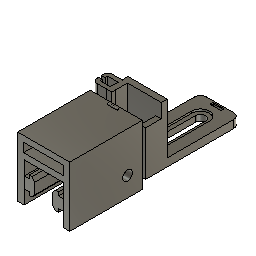
Sensor_Support (Autodesk Fusion 360 design; units mm, degrees)
Autodesk Fusion 360 part; units mm, degrees
sketch "Esquisse1" plane through (0, 0, 0) normal (0, 0, 1) x (1, 0, 0)
  line L0 (0, 80) -> (0, -6.3898) construction
  line L1 (-15, 30) -> (6, 30) construction
  line L2 (-7.25, 0) -> (7.25, 0)
  line L3 (7.25, 0) -> (7.25, -6)
  line L4 (-7.25, -6) -> (-7.25, 0)
  line L5 (-5.5, -1) -> (5.5, -1)
  line L6 (5.5, -1) -> (5.5, -6)
  line L7 (5.5, -6) -> (-5.5, -6)
  line L8 (-5.5, -6) -> (-5.5, -1)
  line L9 (5.5, -6) -> (7.25, -6)
  line L10 (7.25, -6) -> (-5.5, -6)
  line L11 (-7.25, -6) -> (-5.5, -6)
  line L12 (-10, 0) -> (-10, 37)
  line L13 (-7, 40) -> (7, 40)
  arc A0 (4.5, 30) -> (-4.5, 30) centre (0, 30) ccw
  arc A1 (2.5, 30) -> (-2.5, 30) centre (0, 30) ccw
  line L14 (-13, 20) -> (15, 20) construction
  line L15 (-13, 10) -> (15, 10) construction
  arc A2 (-4.5, 10) -> (4.5, 10) centre (0, 10) ccw
  arc A3 (-2.5, 10) -> (2.5, 10) centre (0, 10) ccw
  line L16 (-4.5, 30) -> (-4.5, 10)
  line L17 (-2.5, 30) -> (-2.5, 10)
  line L18 (2.5, 30) -> (2.5, 10)
  line L19 (4.5, 30) -> (4.5, 10)
  line L20 (-19.75, -1.5) -> (-19.75, -9) construction
  line L21 (-15.265, -2) -> (-12, -2)
  line L22 (-10, -8) -> (-14.75, -8)
  line L23 (-14.7654, 0) -> (-10, 0)
  line L24 (-17.25, -3.35) -> (-15.265, -3.35)
  line L25 (-15.25, -4.7238) -> (-17.25, -4.7238)
  line L26 (-15.265, -3.35) -> (-15.265, -2)
  line L27 (-17.25, -5.5) -> (-17.25, -4.7238)
  line L28 (-17.25, -3.35) -> (-17.265, -2.5467)
  arc A4 (-14.7654, 0) -> (-17.265, -2.5467) centre (-14.7654, -2.5) ccw
  arc A5 (-17.25, -5.5) -> (-14.75, -8) centre (-14.75, -5.5) ccw
  line L29 (-12, -2) -> (-10, -2)
  line L30 (-10, -2) -> (-10, -6)
  line L31 (-10, -6) -> (-15.25, -6)
  line L32 (-15.25, -6) -> (-15.25, -4.7238)
  line L33 (-13, -4.0369) -> (-21, -4.0369) construction
  line L34 (10, -8) -> (-10, -8)
  line L35 (10, 37) -> (10, -8)
  line L36 (10, 3) -> (-10, 3)
  arc A6 (-7, 40) -> (-10, 37) centre (-7, 37) ccw
  arc A7 (10, 37) -> (7, 40) centre (7, 37) ccw
  line L37 (-2.5, 39) -> (2.5, 39)
  line L38 (2.5, 39) -> (2.5, 38)
  line L39 (2.5, 38) -> (-2.5, 38)
  line L40 (-2.5, 38) -> (-2.5, 39)
  dimension "d49" = 11
  dimension "d50" = 5
  dimension "d51" = 1
  dimension "d52" = 14.5
  dimension "d67" = 30
  dimension "d68" = 5
  dimension "d86" = 10
  dimension "d87" = 2
  dimension "d100" = 2.5
  dimension "d101" = 2.5
  dimension "d108" = 2
  dimension "d109" = 2
  dimension "d111" = 1.3738
  dimension "d112" = 2
  dimension "d113" = 2
  dimension "d114" = 5.25
  dimension "d115" = 4
  dimension "d117" = 1.2762
  dimension "d132" = 2
  dimension "d133" = 5.265
  dimension "d135" = 48
  dimension "d136" = 20
  dimension "d137" = 2.75
  dimension "d140" = 3
  dimension "d153" = 3
  dimension "d154" = 1
  dimension "d155" = 1
  dimension "d156" = 5
  constraint perpendicular L0 L1
  constraint horizontal L2
  constraint vertical L3
  constraint vertical L4
  constraint symmetric L0 L3 L4
  constraint horizontal L5
  constraint vertical L6
  constraint horizontal L7
  constraint vertical L8
  constraint symmetric L0 L6 L8
  constraint coincident origin L0
  constraint coincident origin L2
  constraint perpendicular L3 L9
  constraint perpendicular L8 L11
  constraint perpendicular L1 L12
  constraint coincident L0 A0.centre
  constraint coincident L1 A0.centre
  constraint concentric A0 A1
  constraint coincident L1 A0.end
  constraint coincident L1 A1.end
  constraint coincident L1 A1.start
  constraint coincident L1 A0.start
  constraint horizontal L14
  constraint perpendicular L12 L15
  constraint symmetric A0.end L14 A2.start
  constraint symmetric A0 L14 A2
  constraint symmetric A1.end L14 A3.start
  constraint symmetric A1 L14 A3
  constraint symmetric A1.start L14 A3.end
  constraint symmetric A0.start L14 A2.end
  constraint horizontal L21
  constraint horizontal L24
  constraint horizontal L25
  constraint coincident L24.start L27
  constraint parallel L21 L23
  constraint tangent L23 A4
  constraint tangent L28 A4
  constraint tangent L27 A5
  constraint tangent L22 A5
  constraint perpendicular L12 L29
  constraint perpendicular L29 L30
  constraint perpendicular L20 L31
  constraint perpendicular L31 L32
  constraint perpendicular L26 L33
  constraint coincident L12.start L23.end
  constraint collinear L12 L30
  constraint vertical L35
  constraint coincident L35 L36.start
  constraint coincident L12 L36.end
  constraint perpendicular L12 L36
  constraint tangent L12 A6
  constraint tangent L13 A6
  constraint tangent L13 A7
  constraint tangent L35 A7
  constraint equal A6 A7
  constraint horizontal L37
  constraint vertical L38
  constraint horizontal L39
  constraint vertical L40
  constraint symmetric L0 L38 L40
  measures "d49" distance of L5.start L5.end
  measures "d50" distance of L5 L7
  measures "d51" distance of L2 L5
  measures "d52" distance of L3 L4
  measures "d67" distance of L1 L2
  measures "d68" diameter of A1
  measures "d86" distance of L2 L15
  measures "d87" distance of L18 L19
  measures "d100" radius of A4
  measures "d101" radius of A5
  measures "d108" distance of L22 L31
  measures "d109" distance of L21 L23
  measures "d111" distance of L24 L25
  measures "d112" distance of L27 L32
  measures "d113" distance of L26 L28.end
  measures "d114" distance of L30 L32
  measures "d115" distance of L21 L31
  measures "d117" distance of L25 L31
  measures "d132" distance of L7 L34
  measures "d133" distance of L26 L30
  measures "d135" distance of L13 L34
  measures "d136" distance of L12 L35
  measures "d137" distance of L4 L12
  measures "d140" distance of L2 L36
  measures "d153" radius of A6
  measures "d154" distance of L37 L39
  measures "d155" distance of L13 L37
  measures "d156" distance of L38 L40
extrude "Extrusion18" add sketch "Esquisse1" along normal blind 2 contours L2 L3 L4 L5 L6 L8 L9 L10 L11 makes body 1
extrude "Extrusion19" add sketch "Esquisse1" along normal blind 4 separate body contours L12 L13 L35 L36 A6 A7 | A0 A2 L16 L19 | L37 L38 L39 L40 makes body 2
extrude "Extrusion20" add sketch "Esquisse1" along normal blind 30 contours L12 L21 L22 L23 L24 L25 L26 L27 L28 A4 A5 L29 L30 L31 L32 L34 L35 L36 bodies 1 2
sketch "Esquisse11" plane through (0, -8, 0) normal (0, -1, 0) x (1, 0, 0)
  line L0 (-10, 0) -> (10, 0)
  line L1 (10, 0) -> (10, 30)
  line L2 (10, 30) -> (-10, 30)
  line L3 (-10, 30) -> (-10, 0)
  line L4 (7.25, 2) -> (7.25, 30)
  line L5 (-7.25, 2) -> (-7.25, 30)
  line L6 (-7.25, 30) -> (-7.25, 16)
  line L7 (-0.45, 16) -> (-0.45, 22.8)
  line L8 (-0.45, 22.8) -> (7.25, 22.8)
  line L9 (-7.25, 16) -> (-0.45, 16)
  dimension "d145" = 6.8
  dimension "d146" = 6.8
  dimension "d147" = 16
  constraint coincident L5.end L6.start
  constraint midpoint L5 L6.end
  constraint perpendicular L2 L7
  constraint coincident L4 L8.end
  constraint perpendicular L4 L8
  constraint coincident L7 L9.end
  constraint perpendicular L7 L9
  constraint coincident L7.start L9.end
  measures "d145" distance of L6 L7
  measures "d146" distance of L8 L9
  measures "d147" distance of L0 L9
extrude "Extrusion21" cut sketch "Esquisse11" against normal up to surface (2 mm away) contours L2 L4 L5 L6 L7 L8 L9 bodies 1
extrude "Extrusion22" cut sketch "Esquisse1" against normal blind 1 from surface at 4 contours A0 A2 L16 L19 bodies 1
copy_body "Corps->Comp1" bodies 1 removing the originals makes body 3 in component "IR_Support"
extrude "Extrusion1" cut sketch "Esquisse1" against normal blind 2 from surface at 4 contours L37 L38 L39 L40 bodies 3 in component "IR_Support"
fillet "Congé1" radius 0.3 4 edges at (2.5, 38.5, 4) (0, 38, 4) (-2.5, 38.5, 4) (0, 39, 4) on bodies 3 in component "IR_Support"
ref_plane "Plan de construction1" through (0, 3, 0) normal (0, 1, 0) x (0, 0, 1) in component "Frame_Support"
sketch "Esquisse1 (2)" plane through (0, 3, 0) normal (0, 1, 0) x (1, 0, 0) in component "Frame_Support"
  line L0 (-10, -4) -> (10, -4)
  line L1 (10, -4) -> (10, 0)
  line L2 (10, 0) -> (-10, 0)
  line L3 (-10, 0) -> (-10, -4)
  line L4 (-10.3, -4.3) -> (10.3, -4.3)
  line L5 (10.3, -4.3) -> (10.3, 0.3)
  line L6 (10.3, 0.3) -> (-10.3, 0.3)
  line L7 (-10.3, 0.3) -> (-10.3, -4.3)
  line L8 (-13.3, -7.3) -> (13.3, -7.3)
  line L9 (13.3, -7.3) -> (13.3, 23.3)
  line L10 (-13.3, 23.3) -> (-13.3, -7.3)
  line L11 (0, -1.75) -> (0, -22.5)
  line L12 (10, 3.3) -> (-10, 3.3)
  line L13 (-10, 23.3) -> (-10, 3.3)
  line L14 (10, 3.3) -> (10, 23.3)
  line L15 (13.3, 23.3) -> (10, 23.3)
  line L16 (-10, 23.3) -> (-13.3, 23.3)
  line L17 (-15, 13.3) -> (16, 13.3) construction
  line L18 (-5.9999, 8.8) -> (-7.4999, 8.8)
  line L19 (-7.4999, 8.8) -> (-7.4999, 10.5)
  line L20 (-7.4999, 10.5) -> (-9.9999, 10.5)
  line L21 (-9.9999, 10.5) -> (-9.9999, 16.1)
  line L22 (-9.9999, 16.1) -> (-7.4999, 16.1)
  line L23 (-7.4999, 16.1) -> (-7.4999, 17.8)
  line L24 (-7.4999, 17.8) -> (-5.9999, 17.8)
  line L25 (-5.9999, 17.8) -> (-4.5028, 16.0546)
  line L26 (-4.5028, 16.0546) -> (-4.5028, 10.4546)
  line L27 (-4.5028, 10.4546) -> (-5.9999, 8.8)
  line L28 (5.9999, 8.8) -> (7.4999, 8.8)
  line L29 (7.4999, 8.8) -> (7.4999, 10.5)
  line L30 (7.4999, 10.5) -> (9.9999, 10.5)
  line L31 (9.9999, 10.5) -> (9.9999, 16.1)
  line L32 (9.9999, 16.1) -> (7.4999, 16.1)
  line L33 (7.4999, 16.1) -> (7.4999, 17.8)
  line L34 (7.4999, 17.8) -> (5.9999, 17.8)
  line L35 (5.9999, 17.8) -> (4.5028, 16.0546)
  line L36 (4.5028, 10.4546) -> (5.9999, 8.8)
  line L37 (4.5028, 16.0546) -> (4.5028, 10.4546)
  dimension "d163" = 20
  dimension "d164" = 4
  dimension "d165" = 0.3
  dimension "d166" = 3
  dimension "d167" = 3
  dimension "d168" = 3
  dimension "d169" = 20
  dimension "d170" = 20
  dimension "d171" = 3.3
  dimension "d17" = 2.5
  dimension "d18" = 2.5
  dimension "d19" = 1.5
  dimension "d20" = 1.5
  dimension "d21" = 5.6
  dimension "d22" = 9
  dimension "d23" = 5.6
  dimension "d26" = 1.7
  constraint horizontal L0
  constraint vertical L1
  constraint horizontal L2
  constraint vertical L3
  constraint horizontal L8
  constraint vertical L9
  constraint horizontal L15
  constraint vertical L10
  constraint symmetric L9 L10 L11
  constraint perpendicular L10 L12
  constraint coincident L13.start L15
  constraint perpendicular L13 L15
  constraint perpendicular L14 L15
  constraint symmetric L11 L13 L14
  constraint collinear L15 L16
  constraint coincident origin L2
  constraint perpendicular L10 L17
  constraint horizontal L22
  constraint perpendicular L22 L23
  constraint perpendicular L23 L24
  constraint perpendicular L24 L26
  constraint perpendicular L18 L26
  constraint perpendicular L18 L19
  constraint perpendicular L20 L26
  constraint perpendicular L21 L22
  constraint symmetric L17 L20 L22
  constraint symmetric L11 L26.end L36.start
  constraint symmetric L11 L20.end L30.end
  constraint symmetric L11 L21.end L31.end
  constraint symmetric L11 L22.end L32.end
  constraint symmetric L11 L18.start L28.start
  constraint symmetric L11 L25.end L35.end
  constraint symmetric L11 L24.end L34.end
  constraint symmetric L11 L23.end L33.end
  constraint symmetric L11 L19.end L29.end
  constraint symmetric L11 L18.end L28.end
  measures "d163" distance of L0.start L0.end
  measures "d164" distance of L0.start L2.end
  measures "d166" distance of L5 L9
  measures "d167" distance of L4 L8
  measures "d168" distance of L6 L12
  measures "d169" distance of L12 L15
  measures "d170" distance of L13 L14
  measures "d171" distance of L9 L14
  measures "d17" distance of L21.end L22.end
  measures "d18" distance of L20.end L19.end
  measures "d19" distance of L18.start L18.end
  measures "d20" distance of L24.end L23.end
  measures "d21" distance of L20 L22
  measures "d22" distance of L18 L24
  measures "d23" distance of L26.end L25.end
  measures "d26" distance of L19.end L18.end
extrude "Extrusion1'" add sketch "Esquisse1 (2)" along normal blind 37 separate body contours L8 L9 L10 L12 L13 L14 L15 L16 L21 L31 makes body 4 in component "Frame_Support"
extrude "Extrusion2" add sketch "Esquisse1 (2)" along normal blind 20 separate body contours L13 L18 L19 L20 L21 L22 L23 L24 L25 L26 L27 | L14 L28 L29 L30 L31 L32 L33 L34 L35 L36 L37 makes body 5 at (-4.5028, 9.6667, -14.188) makes body 6 at (4.5028, 9.6667, -14.188) in component "Frame_Support"
sketch "Esquisse2" plane through (13.3, 0, 0) normal (1, 0, 0) x (0, 1, 0) in component "Frame_Support"
  line L0 (3, 7.3) -> (3, -23.3)
  line L1 (3, -23.3) -> (40, -23.3)
  line L2 (40, -23.3) -> (40, 7.3)
  line L3 (40, 7.3) -> (3, 7.3)
  line L4 (45, -13.3) -> (20, -13.3) construction
  line L5 (32.5, -5) -> (32.5, -27.6162) construction
  circle A0 centre (32.5, -13.3) radius 2.5
  dimension "d184" = 10
  dimension "d185" = 7.5
  dimension "d186" = 5
  constraint perpendicular L2 L4
  constraint perpendicular L1 L5
  constraint midpoint L4 A0.centre
  measures "d184" distance of L1 L4
  measures "d185" distance of L2 L5
  measures "d186" diameter of A0
extrude "Extrusion3" cut sketch "Esquisse2" against normal up to surface (26.6 mm away) contours A0 bodies 4 in component "Frame_Support"
sketch "Esquisse3" plane through (0, 0, 7.3) normal (0, 0, 1) x (-1, 0, 0) in component "Frame_Support"
  line L0 (13.3, -3) -> (-13.3, -3)
  line L1 (-13.3, -3) -> (-13.3, -40)
  line L2 (-13.3, -40) -> (13.3, -40)
  line L3 (13.3, -40) -> (13.3, -3)
  line L4 (20, -38.5) -> (-20, -38.5) construction
  line L5 (2.5, -39) -> (-2.5, -39)
  line L6 (-2.5, -39) -> (-2.5, -38)
  line L7 (-2.5, -38) -> (2.5, -38)
  line L8 (2.5, -38) -> (2.5, -39)
  line L9 (0, -42) -> (0, -32) construction
  line L10 (-13.3, -40) -> (-13.3, -3)
  dimension "d190" = 5
  dimension "d191" = 1
  dimension "d192" = 1
  constraint perpendicular L3 L4
  constraint horizontal L5
  constraint vertical L6
  constraint horizontal L7
  constraint vertical L8
  constraint symmetric L4 L5 L7
  constraint vertical L9
  constraint symmetric L6 L8 L9
  measures "d190" distance of L5.start L5.end
  measures "d191" distance of L5.start L7.end
  measures "d192" distance of L2 L5
extrude "Extrusion4" add sketch "Esquisse3" along normal blind 0.5 contours L5 L6 L7 L8 bodies 4 in component "Frame_Support"
fillet "Congé1'" radius 0.5 2 edges at (0, 38, 7.8) (0, 39, 7.8) on bodies 4 in component "Frame_Support"
sketch "Esquisse3 (2)" plane through (0, 0, 30) normal (0, 0, 1) x (-1, 0, 0) in component "IR_Support"
  line L0 (-7.25, 6) -> (-7.25, 8)
  line L1 (-7.25, 8) -> (-10, 8)
  line L2 (-10, 8) -> (-10, -3)
  line L3 (-10, -3) -> (10, -3)
  line L4 (10, -3) -> (10, 0)
  line L5 (10, 0) -> (14.7654, 0)
  arc A0 (14.7654, 0) -> (17.265, 2.5467) centre (14.7654, 2.5) ccw
  line L6 (17.265, 2.5467) -> (17.25, 3.35)
  line L7 (17.25, 3.35) -> (15.265, 3.35)
  line L8 (15.265, 3.35) -> (15.265, 2)
  line L9 (15.265, 2) -> (10, 2)
  line L10 (10, 2) -> (10, 6)
  line L11 (10, 6) -> (15.25, 6)
  line L12 (15.25, 6) -> (15.25, 4.7238)
  line L13 (15.25, 4.7238) -> (17.25, 4.7238)
  line L14 (17.25, 4.7238) -> (17.25, 5.5)
  arc A1 (17.25, 5.5) -> (14.75, 8) centre (14.75, 5.5) ccw
  line L15 (14.75, 8) -> (10, 8)
  line L16 (10, 8) -> (7.25, 8)
  line L17 (7.25, 8) -> (7.25, 6)
  line L18 (7.25, 6) -> (7.25, 0)
  line L19 (7.25, 0) -> (-7.25, 0)
  line L20 (-7.25, 0) -> (-7.25, 6)
  line L21 (-7.25, 0) -> (-10, 0)
  line L22 (-10, 0) -> (-10, 8)
  line L23 (-10, 8) -> (-7.25, 8)
  line L24 (-7.25, 8) -> (-7.25, 0)
  point P0 (-7.25, 8)
  constraint horizontal L21
  constraint vertical L22
  constraint horizontal L23
  constraint vertical L24
  constraint coincident L24 P0
  constraint coincident L1.end L23
  constraint coincident L19.end L21
  constraint coincident L1.end L22
extrude "Extrusion2'" cut sketch "Esquisse3 (2)" against normal blind 7.2 contours L0 L1 L2 L20 L21 L22 L23 L24 bodies 3 in component "IR_Support"
component "IR_Support" placed x (1, 0, 0) y (0, 1, 0) z (0, 0, 1) at (0, 0, 0)
component "Frame_Support" placed x (1, 0, 0) y (0, 1, 0) z (0, 0, 1) at (0, 0, 0)
